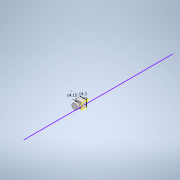
# Autodesk Inventor part: dummy camera
Saved by Autodesk Inventor 2020 (Build 240168000, 168)
## iProperties
Created: 2022-06-22
Part Number: dummy camera
Material: Generic
Document SubType Name: Modeling
Designer: Steven
Density: 1 g/cm^3
Appearance: Default
Author: Steven
Autodesk Inventor part; units mm, degrees
ref_plane "YZ Plane" through (0, 0, 0) normal (1, 0, 0) x (0, 1, 0)
ref_plane "XZ Plane" through (0, 0, 0) normal (0, 1, 0) x (-1, 0, 0)
sketch "Sketch1" plane through (0, 0, 0) normal (0, 0, 1) x (1, 0, 0)
  line L0 (0, 0) -> (-14.3, 0)
  line L1 (-14.3, 0) -> (-14.3, 14.15)
  line L2 (-14.3, 14.15) -> (0, 14.15)
  line L3 (0, 14.15) -> (0, 0)
  dimension "d0" = 14.15
  dimension "d1" = 14.3
  constraints: 8 end point, 2 parallel, 1 horizontal, 1 perpendicular
  measures "d0" distance of L0.end L1.end
  measures "d1" distance of L1.end L2.end
extrude "Extrusion1" add sketch "Sketch1" along normal blind 8
sketch "Sketch2" plane through (0, 0, 0) normal (1, 0, 0) x (0, 0, -1)
  line L0 (0, 0) -> (0, 14.15) projected
  line L1 (0, 14.15) -> (-8, 14.15) projected
  line L2 (-8, 0) -> (-8, 14.15) projected
  line L3 (0, 0) -> (-8, 0) projected
  line L4 (0, 0) -> (0, 14.15) construction
  line L5 (0, 7.075) -> (-10.75, 7.075) construction
  line L6 (-8, 0) -> (-8, 14.15) projected
  circle A0 centre (-8, 7.075) radius 1
  circle A1 centre (-8, 7.075) radius 2.75
  point P0 (-8, 9.825)
  point P1 (-8, 4.325)
  point P2 (-8, 8.075)
  point P3 (-8, 6.075)
  dimension "d4" = 10.75
  dimension "d5" = 2
  constraints: 2 end point, 2 midpoint, 1 centre point, 1 coincident, 1 horizontal, 3 other
  measures "d4" distance of L5.start L5.end
  measures "d5" diameter of A0
extrude "Extrusion2" add sketch "Sketch2" against normal up to surface (14.3 mm away) contours A1 L2 A0 | A0 L2 picked at (-9.5833, 8.5314) picked at (-8.3098, 7.4083)
extrude "Extrusion3" cut sketch "Sketch2" against normal up to surface (14.3 mm away) contours A0 L2 | L2 A0
ref_plane "Work Plane1" through (0, 7.075, 10.75) normal (0, 0, 1) x (1, 0, 0)
sketch "Sketch3" plane through (0, 7.075, 10.75) normal (0, 0, 1) x (1, 0, 0)
  line L0 (-14.3, 2.75) -> (0, 2.75) projected
  line L1 (0, 2.75) -> (0, 7.075) projected
  line L2 (0, 7.075) -> (-14.3, 7.075) projected
  line L3 (-14.3, 7.075) -> (-14.3, 2.75) projected
  line L4 (0, -2.75) -> (-14.3, -2.75) projected
  line L5 (-14.3, -2.75) -> (-14.3, -7.075) projected
  line L6 (-14.3, -7.075) -> (0, -7.075) projected
  line L7 (0, -7.075) -> (0, -2.75) projected
  line L8 (-14.3, 2.75) -> (-14.3, -2.75) projected
  line L9 (0, -2.75) -> (-14.3, -2.75) projected
  line L10 (0, 2.75) -> (0, -2.75) projected
  line L11 (-14.3, 2.75) -> (0, 2.75) projected
  line L12 (0, 7.075) -> (-14.3, 7.075) construction
  line L13 (-7.15, 7.075) -> (-7.15, -7.075) construction
  line L14 (-14.3, -7.075) -> (0, -7.075) construction
  circle A0 centre (-7.15, 0) radius 6.15
  dimension "d10" = 12.3
  constraints: 3 midpoint, 2 end point, 1 centre point
  measures "d10" diameter of A0
extrude "Extrusion4" add sketch "Sketch3" against normal up to surface (2.75 mm away) contours A0 L0 | L0 A0 L4 | L4 A0
extrude "Extrusion5" cut sketch "Sketch2" against normal up to surface (14.3 mm away) contours A0 L2 picked at (-8.3098, 7.4083)
extrude "Extrusion6" add sketch "Sketch3" along normal blind 8 contours A0 L0 | L0 A0 L4 | L4 A0
sketch "Sketch4" plane through (0, 0, 0) normal (1, 0, 0) x (0, 0, -1)
  line L0 (0, 0) -> (0, 14.15) construction
  line L1 (0, 7.075) -> (-14.5, 7.075) construction
  line L2 (-18.75, 0.925) -> (-8, 0.925) construction
  line L3 (-14.5, 0.925) -> (-23.2095, 0.925)
  line L4 (-23.2095, 0.925) -> (-23.2095, 17.6688)
  line L5 (-23.2095, 17.6688) -> (-14.5, 17.6688)
  line L6 (-14.5, 17.6688) -> (-14.5, 0.925)
  dimension "d17" = 14.5
  constraints: 10 end point, 2 horizontal, 2 parallel, 1 midpoint, 1 perpendicular, 1 point on line
  measures "d17" distance of L1.start L1.end
extrude "Extrusion7" cut sketch "Sketch4" against normal through all
sketch "Sketch5" plane through (-7.15, 7.075, 14.5) normal (0, 0, 1) x (1, 0, 0)
  circle A0 centre (0, 0) radius 6.55
  point P0 (7.15, -7.075)
  dimension "d20" = 13.1
  constraints: 1 centre point
  measures "d20" diameter of A0
extrude "Extrusion8" add sketch "Sketch5" along normal blind 8
sketch "Sketch6" plane through (0, 0, 0) normal (1, 0, 0) x (0, 0, -1)
  circle A0 centre (-8, 7.075) radius 1 construction
  line L0 (0, 0) -> (0, 14.15) construction
  line L1 (0, 14.15) -> (-8, 14.15) construction
  line L2 (-8, 9.825) -> (-8, 14.15) construction
  arc A1 (-8, 9.825) -> (-8, 4.325) centre (-8, 7.075) ccw construction
  line L3 (-8, 0) -> (-8, 4.325) construction
  line L4 (0, 0) -> (-8, 0) construction
  line L5 (0, 14.15) -> (0, 0) construction
  line L6 (0, 7.075) -> (-19.3, 7.075) construction
  line L7 (-14.5, 0.525) -> (-22.5, 0.525) projected
  line L8 (-19.3, 0.525) -> (-27.8316, 0.525)
  line L9 (-27.8316, 0.525) -> (-27.8316, 15.7859)
  line L10 (-27.8316, 15.7859) -> (-19.3, 15.7859)
  line L11 (-19.3, 15.7859) -> (-19.3, 0.525)
  dimension "d23" = 19.3
  constraints: 10 end point, 2 horizontal, 2 parallel, 1 midpoint, 1 perpendicular, 1 point on line
  measures "d23" distance of L6.start L6.end
extrude "Extrusion9" cut sketch "Sketch6" against normal through all
fillet "Fillet1" radius 5 4 edges at (-0.8245, 4.325, 8) (-0.8245, 9.825, 8) (-13.4755, 4.325, 8) (-13.4755, 9.825, 8)
sketch "Sketch7" plane through (0, 0, 0) normal (0, 0, -1) x (-1, 0, 0)
  line L0 (14.3, 0) -> (0, 0) projected
  line L1 (14.3, 14.15) -> (14.3, 0) projected
  line L2 (0, 14.15) -> (14.3, 14.15) projected
  line L3 (0, 0) -> (0, 14.15) projected
  line L4 (0, 14.15) -> (14.3, 14.15) projected
  line L5 (0, 14.15) -> (8.35, 14.15)
  line L6 (8.35, 14.15) -> (8.35, 10.7)
  line L7 (8.35, 10.7) -> (0, 10.7)
  line L8 (0, 10.7) -> (0, 14.15)
  dimension "d28" = 8.35
  dimension "d29" = 3.45
  constraints: 8 end point, 2 parallel, 1 horizontal, 1 perpendicular
  measures "d28" distance of L6.end L7.end
  measures "d29" distance of L5.end L6.end
extrude "Extrusion10" add sketch "Sketch7" along normal blind 3.55 contours L3 L2 L6 L7
sketch "Sketch8" plane through (0, 7.075, 10.75) normal (0, 0, 1) x (1, 0, 0)
  line L0 (0, 7.075) -> (-14.3, 7.075) projected
  line L1 (-14.3, -7.075) -> (0, -7.075) projected
  line L2 (-14.3, 7.075) -> (-14.3, -7.075)
  line L3 (0, -7.075) -> (0, 7.075)
  constraints: 4 end point, 1 parallel, 1 vertical
extrude "Extrusion11" add sketch "Sketch8" against normal up to surface (2.75 mm away)
extrude "Extrusion12" cut sketch "Sketch2" against normal up to surface (14.3 mm away) contours A0 L2 picked at (-8.3098, 7.4083)
sketch "Sketch9" plane through (0, 0, 0) normal (1, 0, 0) x (0, 0, -1)
  circle A0 centre (-8, 7.075) radius 1 projected
  line L0 (0, 0) -> (-10.75, 0) projected
  line L1 (0, 0) -> (0, 10.7) projected
  line L2 (0, 10.7) -> (3.55, 10.7) projected
  line L3 (3.55, 14.15) -> (3.55, 10.7) projected
  line L4 (3.55, 14.15) -> (-10.75, 14.15) projected
  line L5 (-10.75, 0) -> (-10.75, 14.15) projected
  line L6 (0, 7.075) -> (-142.5994, 7.075)
  line L7 (0, 7.075) -> (195.5312, 7.075)
  constraints: 4 end point, 1 collinear, 1 horizontal, 1 point on line
body "Solid1"
